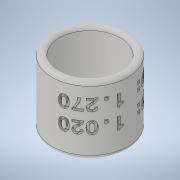
# Autodesk Inventor part: LargeFinderEyePieceCover
Saved by Autodesk Inventor 2021.1 (Build 251245000, 245)
## iProperties
Created: 2018-09-01
Part Number: LargeFinderEyePieceCover
Material: Generic
Document SubType Name: Modeling
Designer: steele
Density: 1 g/cm^3
Appearance: Default
Author: steele
Autodesk Inventor part; units mm, degrees
ref_plane "XZ Plane" through (0, 0, 0) normal (0, 1, 0) x (-1, 0, 0)
ref_plane "XY Plane" through (0, 0, 0) normal (0, 0, 1) x (1, 0, 0)
sketch "Sketch1" plane through (0, 0, 0) normal (0, 1, 0) x (-1, 0, 0)
  circle A0 centre (0, 0) radius 16.129
  dimension "d0" = 32.258
  constraints: 1 centre point, 1 coincident
  measures "d0" diameter of A0
extrude "Extrusion1" add sketch "Sketch1" along normal blind 3.175
sketch "Sketch2" plane through (0, 3.175, 0) normal (0, 1, 0) x (1, 0, 0)
  circle A0 centre (0, 0) radius 16.129
  circle A1 centre (0, 0) radius 12.954
  dimension "d3" = 32.258
  dimension "d4" = 25.908
  constraints: 2 centre point, 2 coincident
  measures "d3" diameter of A0
  measures "d4" diameter of A1
extrude "Extrusion2" add sketch "Sketch2" along normal blind 25.4
ref_plane "Work Plane1" through (16.129, 0, 0) normal (1, 0, 0) x (0, 1, 0)
sketch "Sketch3" plane through (16.129, 0, 0) normal (1, 0, 0) x (0, 1, 0)
  line L0 (0, 16.129) -> (28.575, 16.129) construction
  line L1 (14.2875, 16.129) -> (14.2875, -16.6287) construction
  line L2 (3.175, -12.954) -> (28.575, -12.954) construction
  line L3 (10.082, -14.961) -> (10.082, -15.8913)
  line L4 (10.082, -15.8913) -> (9.2075, -15.8913)
  line L5 (9.2075, -15.8913) -> (9.2075, -12.9633)
  line L6 (9.2075, -12.9633) -> (10.082, -12.9633)
  line L7 (10.082, -12.9633) -> (10.082, -13.8936)
  line L8 (10.082, -13.8936) -> (13.4087, -13.8936)
  line L9 (13.4087, -13.8936) -> (13.4087, -12.9633)
  line L10 (13.4087, -12.9633) -> (14.2875, -12.9633)
  line L11 (14.2875, -12.9633) -> (14.2875, -15.8913)
  line L12 (14.2875, -15.8913) -> (13.4087, -15.8913)
  line L13 (13.4087, -15.8913) -> (13.4087, -14.961)
  line L14 (13.4087, -14.961) -> (10.082, -14.961)
  spline S0 degree 2 poles (9.2075, -10.0182) (9.2075, -9.0923) (10.5021, -8.1277) (11.7454, -8.1277) knots 0 0 0 1 2 2 2
  spline S1 degree 2 poles (11.7454, -8.1277) (13.0057, -8.1277) (14.2875, -9.0837) (14.2875, -10.0182) knots 0 0 0 1 2 2 2
  line L15 (14.2875, -10.0182) -> (14.2875, -11.7116)
  line L16 (14.2875, -11.7116) -> (9.2075, -11.7116)
  line L17 (9.2075, -11.7116) -> (9.2075, -10.0182)
  line L18 (10.1506, -10.0182) -> (10.1506, -10.6355)
  line L19 (10.1506, -10.6355) -> (13.3358, -10.6355)
  line L20 (13.3358, -10.6355) -> (13.3358, -10.0182)
  spline S2 degree 2 poles (13.3358, -10.0182) (13.3358, -9.6024) (12.5942, -9.2251) (11.7454, -9.2251) knots 0 0 0 1 2 2 2
  spline S3 degree 2 poles (11.7454, -9.2251) (10.9566, -9.2251) (10.1506, -9.6281) (10.1506, -10.0182) knots 0 0 0 1 2 2 2
  line L21 (12.9414, -6.2757) -> (12.9414, -4.9297)
  line L22 (12.9414, -4.9297) -> (14.2875, -4.9297)
  line L23 (14.2875, -4.9297) -> (14.2875, -6.2757)
  line L24 (14.2875, -6.2757) -> (12.9414, -6.2757)
  line L25 (10.3564, -6.2757) -> (10.3564, -4.9297)
  line L26 (10.3564, -4.9297) -> (11.7025, -4.9297)
  line L27 (11.7025, -4.9297) -> (11.7025, -6.2757)
  line L28 (11.7025, -6.2757) -> (10.3564, -6.2757)
  line L29 (10.7894, 3.014) -> (10.7894, 1.7922)
  line L30 (10.7894, 1.7922) -> (10.0692, 1.7922)
  line L31 (10.0692, 1.7922) -> (10.0692, 1.8437)
  spline S4 degree 2 poles (10.0692, 1.8437) (10.0692, 2.5467) (9.6705, 3.1426) (9.1689, 3.2026) knots 0 0 0 1 2 2 2
  line L32 (9.1689, 3.2026) -> (9.1689, 4.0257)
  line L33 (9.1689, 4.0257) -> (14.2875, 4.0257)
  line L34 (14.2875, 4.0257) -> (14.2875, 3.014)
  line L35 (14.2875, 3.014) -> (10.7894, 3.014)
  line L36 (12.9414, 6.958) -> (12.9414, 8.3041)
  line L37 (12.9414, 8.3041) -> (14.2875, 8.3041)
  line L38 (14.2875, 8.3041) -> (14.2875, 6.958)
  line L39 (14.2875, 6.958) -> (12.9414, 6.958)
  spline S5 degree 2 poles (11.7325, 10.1903) (10.4721, 10.1903) (9.1689, 11.1291) (9.1689, 12.0423) knots 0 0 0 1 2 2 2
  spline S6 degree 2 poles (9.1689, 12.0423) (9.1689, 12.9682) (10.485, 13.8899) (11.8097, 13.8899) knots 0 0 0 1 2 2 2
  spline S7 degree 2 poles (11.8097, 13.8899) (13.13, 13.8899) (14.429, 12.9768) (14.429, 12.0423) knots 0 0 0 1 2 2 2
  spline S8 degree 2 poles (14.429, 12.0423) (14.429, 11.1034) (13.1043, 10.1903) (11.7325, 10.1903) knots 0 0 0 1 2 2 2
  spline S9 degree 2 poles (10.0263, 12.0337) (10.0263, 11.635) (10.8623, 11.2535) (11.7368, 11.2535) knots 0 0 0 1 2 2 2
  spline S10 degree 2 poles (11.7368, 11.2535) (12.7185, 11.2535) (13.5759, 11.6221) (13.5759, 12.0337) knots 0 0 0 1 2 2 2
  spline S11 degree 2 poles (13.5759, 12.0337) (13.5759, 12.4452) (12.7271, 12.8268) (11.8011, 12.8268) knots 0 0 0 1 2 2 2
  spline S12 degree 2 poles (11.8011, 12.8268) (10.8708, 12.8268) (10.0263, 12.4452) (10.0263, 12.0337) knots 0 0 0 1 2 2 2
  line L40 (10.9994, 15.6176) -> (10.9994, 14.6744)
  line L41 (10.9994, 14.6744) -> (10.978, 14.6744)
  spline S13 degree 2 poles (10.978, 14.6744) (10.1335, 14.6744) (9.1689, 15.6133) (9.1689, 16.4364) knots 0 0 0 1 2 2 2
  spline S14 degree 2 poles (9.1689, 16.4364) (9.1689, 17.268) (10.022, 18.2326) (10.7422, 18.2326) knots 0 0 0 1 2 2 2
  spline S15 degree 2 poles (10.7422, 18.2326) (11.2566, 18.2326) (12.024, 17.7267) (12.4827, 17.0237) knots 0 0 0 1 2 2 2
  spline S16 degree 2 poles (12.4827, 17.0237) (12.5813, 16.8822) (12.7399, 16.6293) knots 0 0 0 1 1 1
  spline S17 degree 2 poles (12.7399, 16.6293) (13.1815, 15.9348) (13.413, 15.8533) knots 0 0 0 1 1 1
  line L42 (13.413, 15.8533) -> (13.413, 18.1811)
  line L43 (13.413, 18.1811) -> (14.2875, 18.1811)
  line L44 (14.2875, 18.1811) -> (14.2875, 14.5887)
  spline S18 degree 2 poles (14.2875, 14.5887) (13.5887, 14.6016) (12.6499, 15.1674) (12.1569, 15.9005) knots 0 0 0 1 2 2 2
  spline S19 degree 2 poles (12.1569, 15.9005) (12.0797, 16.012) (11.9426, 16.2263) knots 0 0 0 1 1 1
  spline S20 degree 2 poles (11.9426, 16.2263) (11.3338, 17.1866) (10.7594, 17.1866) knots 0 0 0 1 1 1
  spline S21 degree 2 poles (10.7594, 17.1866) (10.425, 17.1866) (10.0263, 16.775) (10.0263, 16.4235) knots 0 0 0 1 2 2 2
  spline S22 degree 2 poles (10.0263, 16.4235) (10.0263, 16.042) (10.5107, 15.6176) (10.9566, 15.6176) knots 0 0 0 1 2 2 2
  line L45 (10.9566, 15.6176) -> (10.9994, 15.6176)
  spline S23 degree 2 poles (11.7325, 19.0128) (10.4721, 19.0128) (9.1689, 19.9516) (9.1689, 20.8647) knots 0 0 0 1 2 2 2
  spline S24 degree 2 poles (9.1689, 20.8647) (9.1689, 21.7907) (10.485, 22.7124) (11.8097, 22.7124) knots 0 0 0 1 2 2 2
  spline S25 degree 2 poles (11.8097, 22.7124) (13.13, 22.7124) (14.429, 21.7993) (14.429, 20.8647) knots 0 0 0 1 2 2 2
  spline S26 degree 2 poles (14.429, 20.8647) (14.429, 19.9259) (13.1043, 19.0128) (11.7325, 19.0128) knots 0 0 0 1 2 2 2
  spline S27 degree 2 poles (10.0263, 20.8562) (10.0263, 20.4575) (10.8623, 20.076) (11.7368, 20.076) knots 0 0 0 1 2 2 2
  spline S28 degree 2 poles (11.7368, 20.076) (12.7185, 20.076) (13.5759, 20.4446) (13.5759, 20.8562) knots 0 0 0 1 2 2 2
  spline S29 degree 2 poles (13.5759, 20.8562) (13.5759, 21.2677) (12.7271, 21.6493) (11.8011, 21.6493) knots 0 0 0 1 2 2 2
  spline S30 degree 2 poles (11.8011, 21.6493) (10.8708, 21.6493) (10.0263, 21.2677) (10.0263, 20.8562) knots 0 0 0 1 2 2 2
  spline S31 degree 2 poles (20.1171, -16.3071) (18.8997, -16.3071) (17.4893, -15.2911) (17.4893, -14.4252) knots 0 0 0 1 2 2 2
  spline S32 degree 2 poles (17.4893, -14.4252) (17.4893, -13.5464) (18.9168, -12.5432) (20.1686, -12.5432) knots 0 0 0 1 2 2 2
  spline S33 degree 2 poles (20.1686, -12.5432) (21.4247, -12.5432) (22.8522, -13.5464) (22.8522, -14.4252) knots 0 0 0 1 2 2 2
  spline S34 degree 2 poles (22.8522, -14.4252) (22.8522, -15.3126) (21.4161, -16.3071) (20.1171, -16.3071) knots 0 0 0 1 2 2 2
  spline S35 degree 2 poles (18.4324, -14.4295) (18.4324, -14.8024) (19.2726, -15.2183) (20.0443, -15.2183) knots 0 0 0 1 2 2 2
  spline S36 degree 2 poles (20.0443, -15.2183) (21.0003, -15.2183) (21.8919, -14.8282) (21.8919, -14.408) knots 0 0 0 1 2 2 2
  spline S37 degree 2 poles (21.8919, -14.408) (21.8919, -14.0179) (21.0646, -13.6407) (20.1814, -13.6407) knots 0 0 0 1 2 2 2
  spline S38 degree 2 poles (20.1814, -13.6407) (19.2983, -13.6407) (18.4324, -14.0308) (18.4324, -14.4295) knots 0 0 0 1 2 2 2
  spline S39 degree 2 poles (17.6307, -10.0182) (17.6307, -9.0923) (18.9254, -8.1277) (20.1686, -8.1277) knots 0 0 0 1 2 2 2
  spline S40 degree 2 poles (20.1686, -8.1277) (21.4289, -8.1277) (22.7107, -9.0837) (22.7107, -10.0182) knots 0 0 0 1 2 2 2
  line L46 (22.7107, -10.0182) -> (22.7107, -11.7116)
  line L47 (22.7107, -11.7116) -> (17.6307, -11.7116)
  line L48 (17.6307, -11.7116) -> (17.6307, -10.0182)
  line L49 (18.5739, -10.0182) -> (18.5739, -10.6355)
  line L50 (18.5739, -10.6355) -> (21.759, -10.6355)
  line L51 (21.759, -10.6355) -> (21.759, -10.0182)
  spline S41 degree 2 poles (21.759, -10.0182) (21.759, -9.6024) (21.0174, -9.2251) (20.1686, -9.2251) knots 0 0 0 1 2 2 2
  spline S42 degree 2 poles (20.1686, -9.2251) (19.3798, -9.2251) (18.5739, -9.6281) (18.5739, -10.0182) knots 0 0 0 1 2 2 2
  line L52 (18.7796, -6.2757) -> (18.7796, -4.9297)
  line L53 (18.7796, -4.9297) -> (20.1257, -4.9297)
  line L54 (20.1257, -4.9297) -> (20.1257, -6.2757)
  line L55 (20.1257, -6.2757) -> (18.7796, -6.2757)
  line L56 (21.3646, -6.2757) -> (21.3646, -4.9297)
  line L57 (21.3646, -4.9297) -> (22.7107, -4.9297)
  line L58 (22.7107, -4.9297) -> (22.7107, -6.2757)
  line L59 (22.7107, -6.2757) -> (21.3646, -6.2757)
  line L60 (19.2126, 3.014) -> (19.2126, 1.7922)
  line L61 (19.2126, 1.7922) -> (18.4924, 1.7922)
  line L62 (18.4924, 1.7922) -> (18.4924, 1.8437)
  spline S43 degree 2 poles (18.4924, 1.8437) (18.4924, 2.5467) (18.0937, 3.1426) (17.5921, 3.2026) knots 0 0 0 1 2 2 2
  line L63 (17.5921, 3.2026) -> (17.5921, 4.0257)
  line L64 (17.5921, 4.0257) -> (22.7107, 4.0257)
  line L65 (22.7107, 4.0257) -> (22.7107, 3.014)
  line L66 (22.7107, 3.014) -> (19.2126, 3.014)
  line L67 (21.3646, 6.958) -> (21.3646, 8.3041)
  line L68 (21.3646, 8.3041) -> (22.7107, 8.3041)
  line L69 (22.7107, 8.3041) -> (22.7107, 6.958)
  line L70 (22.7107, 6.958) -> (21.3646, 6.958)
  line L71 (19.4227, 11.2063) -> (19.4227, 10.2632)
  line L72 (19.4227, 10.2632) -> (19.4012, 10.2632)
  spline S44 degree 2 poles (19.4012, 10.2632) (18.5567, 10.2632) (17.5921, 11.202) (17.5921, 12.0251) knots 0 0 0 1 2 2 2
  spline S45 degree 2 poles (17.5921, 12.0251) (17.5921, 12.8568) (18.4452, 13.8213) (19.1654, 13.8213) knots 0 0 0 1 2 2 2
  spline S46 degree 2 poles (19.1654, 13.8213) (19.6799, 13.8213) (20.4472, 13.3155) (20.9059, 12.6124) knots 0 0 0 1 2 2 2
  spline S47 degree 2 poles (20.9059, 12.6124) (21.0045, 12.471) (21.1632, 12.218) knots 0 0 0 1 1 1
  spline S48 degree 2 poles (21.1632, 12.218) (21.6047, 11.5235) (21.8362, 11.4421) knots 0 0 0 1 1 1
  line L73 (21.8362, 11.4421) -> (21.8362, 13.7699)
  line L74 (21.8362, 13.7699) -> (22.7107, 13.7699)
  line L75 (22.7107, 13.7699) -> (22.7107, 10.1775)
  spline S49 degree 2 poles (22.7107, 10.1775) (22.012, 10.1903) (21.0731, 10.7562) (20.5801, 11.4893) knots 0 0 0 1 2 2 2
  spline S50 degree 2 poles (20.5801, 11.4893) (20.503, 11.6007) (20.3658, 11.8151) knots 0 0 0 1 1 1
  spline S51 degree 2 poles (20.3658, 11.8151) (19.757, 12.7753) (19.1826, 12.7753) knots 0 0 0 1 1 1
  spline S52 degree 2 poles (19.1826, 12.7753) (18.8482, 12.7753) (18.4495, 12.3638) (18.4495, 12.0123) knots 0 0 0 1 2 2 2
  spline S53 degree 2 poles (18.4495, 12.0123) (18.4495, 11.6307) (18.934, 11.2063) (19.3798, 11.2063) knots 0 0 0 1 2 2 2
  line L76 (19.3798, 11.2063) -> (19.4227, 11.2063)
  spline S54 degree 2 poles (22.7107, 15.3475) (21.669, 15.4032) (19.607, 16.3035) (18.6124, 17.1351) knots 0 0 0 1 2 2 2
  line L77 (18.6124, 17.1351) -> (18.6124, 14.6144)
  line L78 (18.6124, 14.6144) -> (17.7379, 14.6144)
  line L79 (17.7379, 14.6144) -> (17.7379, 18.2454)
  line L80 (17.7379, 18.2454) -> (18.5095, 18.2454)
  spline S55 degree 2 poles (18.5095, 18.2454) (19.4527, 17.3966) (21.5018, 16.4964) (22.7107, 16.4106) knots 0 0 0 1 2 2 2
  line L81 (22.7107, 16.4106) -> (22.7107, 15.3475)
  spline S56 degree 2 poles (20.1557, 19.0128) (18.8954, 19.0128) (17.5921, 19.9516) (17.5921, 20.8647) knots 0 0 0 1 2 2 2
  spline S57 degree 2 poles (17.5921, 20.8647) (17.5921, 21.7907) (18.9082, 22.7124) (20.2329, 22.7124) knots 0 0 0 1 2 2 2
  spline S58 degree 2 poles (20.2329, 22.7124) (21.5533, 22.7124) (22.8522, 21.7993) (22.8522, 20.8647) knots 0 0 0 1 2 2 2
  spline S59 degree 2 poles (22.8522, 20.8647) (22.8522, 19.9259) (21.5275, 19.0128) (20.1557, 19.0128) knots 0 0 0 1 2 2 2
  spline S60 degree 2 poles (18.4495, 20.8562) (18.4495, 20.4575) (19.2855, 20.076) (20.16, 20.076) knots 0 0 0 1 2 2 2
  spline S61 degree 2 poles (20.16, 20.076) (21.1417, 20.076) (21.9991, 20.4446) (21.9991, 20.8562) knots 0 0 0 1 2 2 2
  spline S62 degree 2 poles (21.9991, 20.8562) (21.9991, 21.2677) (21.1503, 21.6493) (20.2243, 21.6493) knots 0 0 0 1 2 2 2
  spline S63 degree 2 poles (20.2243, 21.6493) (19.2941, 21.6493) (18.4495, 21.2677) (18.4495, 20.8562) knots 0 0 0 1 2 2 2
  point P0 (0, 0)
  constraints: 2 end point, 1 midpoint, 1 perpendicular, 1 vertical
emboss "Emboss1" sketch "Sketch3" operation cut depth 1.27 direction (1, 0, 0) wrap yes faces at (-15.9201, 10.5833, -2.5873)
fillet "Fillet1" radius 1.5875 1 edges at (16.129, 0, 0)
fillet "Fillet2" radius 1.5875 2 edges at (-12.954, 28.575, 0) (-16.129, 28.575, 0)
equation "\"d0\" = coverOD"
equation "\"d1\" = wallThickness"
equation "\"d3\" = coverOD"
equation "\"d4\" = eypPieceCoverID"
equation "\"d7\" = textDepth"
equation "\"d9\" = filletRadius"
equation "\"d10\" = filletRadius"
equation "\"wallThickness\" = 3.175"
equation "\"coverOD\" = eypPieceCoverID + 2 * wallThickness"
equation "\"eypPieceCoverID\" = 25.908"
equation "\"textDepth\" = 1.27"
equation "\"filletRadius\" = 1.5875"
body "Solid1"
